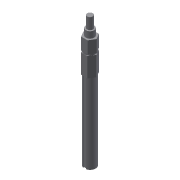
# Autodesk Inventor part: Shaft
Saved by Autodesk Inventor 2015 (Build 190159000, 159)
## iProperties
Created: 2013-02-16
Part Number: Shaft
Material: Generic
Document SubType Name: Modeling
Designer: Tanner
Density: 1 g/cm^3
Appearance: Default
Author: Tanner
Autodesk Inventor part; units mm, degrees
ref_plane "YZ Plane" through (0, 0, 0) normal (1, 0, 0) x (0, 1, 0)
ref_plane "XZ Plane" through (0, 0, 0) normal (0, 1, 0) x (-1, 0, 0)
ref_plane "XY Plane" through (0, 0, 0) normal (0, 0, 1) x (1, 0, 0)
sketch "Sketch1" plane through (0, 0, 0) normal (0, 1, 0) x (-1, 0, 0)
  circle A0 centre (0, 0) radius 6.35
  dimension "d0" = 12.7
  constraints: 1 centre point, 1 coincident
  measures "d0" diameter of A0
extrude "Extrusion1" add sketch "Sketch1" along normal mid plane 88.9
sketch "Sketch2" plane through (0, 44.45, 0) normal (0, 1, 0) x (1, 0, 0)
  circle A0 centre (0, 0) radius 6.35 projected
  line L0 (3.8092, 6.2652) -> (7.3305, -0.1662)
  line L1 (7.3305, -0.1662) -> (3.5213, -6.4315)
  line L2 (3.5213, -6.4315) -> (-3.8092, -6.2652)
  line L3 (-3.8092, -6.2652) -> (-7.3305, 0.1662)
  line L4 (-7.3305, 0.1662) -> (-3.5213, 6.4315)
  line L5 (-3.5213, 6.4315) -> (3.8092, 6.2652)
  dimension "d4" = 12.7
  constraints: 12 end point, 1 coincident, 13 other
  measures "d4" distance between parallel lines of L3 L0
extrude "Extrusion2" add sketch "Sketch2" along normal blind 21.59
sketch "Sketch3" plane through (0, 66.04, 0) normal (0, 1, 0) x (1, 0, 0)
  circle A0 centre (0, 0) radius 6.35
  dimension "d7" = 12.7
  constraints: 1 centre point, 1 coincident
  measures "d7" diameter of A0
extrude "Extrusion3" add sketch "Sketch3" along normal blind 1.778
sketch "Sketch4" plane through (0, 67.818, 0) normal (0, 1, 0) x (1, 0, 0)
  circle A0 centre (0, 0) radius 6.35 projected
  line L0 (7.3323, 0) -> (3.6662, -6.35)
  line L1 (3.6662, -6.35) -> (-3.6662, -6.35)
  line L2 (-3.6662, -6.35) -> (-7.3323, 0)
  line L3 (-7.3323, 0) -> (-3.6662, 6.35)
  line L4 (-3.6662, 6.35) -> (3.6662, 6.35)
  line L5 (3.6662, 6.35) -> (7.3323, 0)
  dimension "d10" = 12.7
  constraints: 12 end point, 1 coincident, 13 other
  measures "d10" distance between parallel lines of L2 L5
extrude "Extrusion4" add sketch "Sketch4" along normal blind 13.462
sketch "Sketch5" plane through (0, 81.28, 0) normal (0, 1, 0) x (1, 0, 0)
  circle A0 centre (0, 0) radius 4.699
  dimension "d13" = 9.398
  constraints: 1 centre point, 1 coincident
  measures "d13" diameter of A0
extrude "Extrusion5" add sketch "Sketch5" along normal blind 7.112
sketch "Sketch6" plane through (0, 88.392, 0) normal (0, 1, 0) x (1, 0, 0)
  circle A0 centre (0, 0) radius 4.699 projected
  circle A1 centre (0, 0) radius 3.2258
  dimension "d16" = 6.4516
  constraints: 1 centre point, 1 coincident
  measures "d16" diameter of A1
extrude "Extrusion6" add sketch "Sketch6" along normal blind 12.7 contours A1
fillet "Fillet1" radius 0.3175 1 edges at (-3.2258, 101.092, 0)
sketch "Sketch7" plane through (0, -44.45, 0) normal (0, -1, 0) x (1, 0, 0)
  line L0 (-1.5875, 6.8356) -> (1.5875, 6.8356)
  line L1 (1.5875, 6.8356) -> (1.5875, 5.0371)
  line L2 (1.5875, 5.0371) -> (-1.5875, 5.0371)
  line L3 (-1.5875, 5.0371) -> (-1.5875, 6.8356)
  line L4 (0, 11.7561) -> (0, 9.7432)
  line L5 (-3.323, -0.0429) -> (4.4977, -0.0429)
  dimension "d20" = 3.175
  dimension "d24" = 5.08
  constraints: 12 end point, 2 parallel, 2 perpendicular, 1 horizontal
  measures "d20" distance between parallel lines of L3 L1
  measures "d24" distance between parallel lines of L5 L2
extrude "Extrusion7" cut sketch "Sketch7" against normal blind 88.9
sketch "Sketch8" plane through (0, -44.45, 0) normal (0, -1, 0) x (1, 0, 0)
  arc A0 (-1.5875, 6.1484) -> (1.5875, 6.1484) centre (0, 0) ccw projected
  circle A1 centre (0, 0) radius 2.032
  dimension "d27" = 4.064
  constraints: 1 centre point, 1 coincident
  measures "d27" diameter of A1
extrude "Extrusion8" cut sketch "Sketch8" against normal blind 50.8
body "Solid1"
